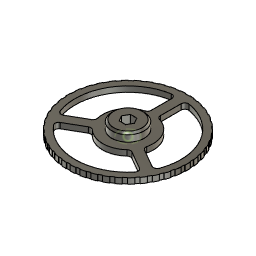
Flange gear v6 (Autodesk Fusion 360 design; units mm, degrees)
description: Spur Gear; Module: 2.0; Num Teeth: 10; Pressure Angle: 20.0; Backlash: 0.00 mm
Autodesk Fusion 360 part; units mm, degrees
(part 1 of 2)
sketch "Sketch1" plane through (0, 0, 0) normal (0, 0, 1) x (1, 0, 0) in component "Spur Gear (10 teeth)"
  circle A0 centre (0, 0) radius 7.5492
extrude "Extrude1" add sketch "Sketch1" along normal blind 7 makes body 1 in component "Spur Gear (10 teeth)"
sketch "Sketch2" plane through (0, 0, 0) normal (0, 0, 1) x (1, 0, 0) in component "Spur Gear (10 teeth)"
  spline S0 degree 5 poles (9.2583, -1.6082) (9.2659, -1.6095) (9.2813, -1.6119) (9.3043, -1.6147) (9.3352, -1.6169) (9.374, -1.6176) (9.4131, -1.6169) (9.4522, -1.6153) (9.4913, -1.6131) (9.5306, -1.6106) (9.5699, -1.6078) (9.6092, -1.6044) (9.6485, -1.6005) (9.688, -1.5957) (9.7275, -1.5903) (9.767, -1.5842) (9.8065, -1.5774) (9.8461, -1.5702) (9.8857, -1.5626) (9.9253, -1.5546) (9.9649, -1.5461) (10.0045, -1.5372) (10.0441, -1.5278) (10.0838, -1.5179) (10.1234, -1.5076) (10.163, -1.4969) (10.2027, -1.4857) (10.2423, -1.4741) (10.2819, -1.4621) (10.3215, -1.4497) (10.3611, -1.4369) (10.4006, -1.4237) (10.4402, -1.4102) (10.4797, -1.3962) (10.5192, -1.3819) (10.5587, -1.3672) (10.5982, -1.3521) (10.6376, -1.3367) (10.677, -1.3209) (10.7163, -1.3047) (10.7557, -1.2882) (10.795, -1.2713) (10.8342, -1.2541) (10.8734, -1.2366) (10.9126, -1.2187) (10.9517, -1.2004) (10.9908, -1.1818) (11.0298, -1.1629) (11.0688, -1.1437) (11.1078, -1.1241) (11.1466, -1.1042) (11.1855, -1.084) (11.2242, -1.0634) (11.2629, -1.0425) (11.3016, -1.0213) (11.3402, -0.9998) (11.3787, -0.978) (11.4172, -0.9559) (11.4556, -0.9334) (11.4939, -0.9107) (11.5322, -0.8876) (11.5704, -0.8642) (11.6085, -0.8406) (11.6466, -0.8166) (11.6846, -0.7923) (11.7225, -0.7677) (11.7603, -0.7429) (11.7981, -0.7177) (11.8358, -0.6923) (11.8733, -0.6665) (11.9109, -0.6405) (11.9408, -0.6194) (11.9632, -0.6035) (11.9781, -0.5928) (11.9856, -0.5875) knots 0 0 0 0 0 0 0.01428571 0.02857143 0.04285714 0.05714286 0.07142857 0.08571429 0.1 0.11428571 0.12857143 0.14285714 0.15714286 0.17142857 0.18571429 0.2 0.21428571 0.22857143 0.24285714 0.25714286 0.27142857 0.28571429 0.3 0.31428571 0.32857143 0.34285714 0.35714286 0.37142857 0.38571429 0.4 0.41428571 0.42857143 0.44285714 0.45714286 0.47142857 0.48571429 0.5 0.51428571 0.52857143 0.54285714 0.55714286 0.57142857 0.58571429 0.6 0.61428571 0.62857143 0.64285714 0.65714286 0.67142857 0.68571429 0.7 0.71428571 0.72857143 0.74285714 0.75714286 0.77142857 0.78571429 0.8 0.81428571 0.82857143 0.84285714 0.85714286 0.87142857 0.88571429 0.9 0.91428571 0.92857143 0.94285714 0.95714286 0.97142857 0.98571429 1 1 1 1 1 1
  spline S1 degree 5 poles (9.2583, 1.6082) (9.2659, 1.6095) (9.2813, 1.6119) (9.3043, 1.6147) (9.3352, 1.6169) (9.374, 1.6176) (9.4131, 1.6169) (9.4522, 1.6153) (9.4913, 1.6131) (9.5306, 1.6106) (9.5699, 1.6078) (9.6092, 1.6044) (9.6485, 1.6005) (9.688, 1.5957) (9.7275, 1.5903) (9.767, 1.5842) (9.8065, 1.5774) (9.8461, 1.5702) (9.8857, 1.5626) (9.9253, 1.5546) (9.9649, 1.5461) (10.0045, 1.5372) (10.0441, 1.5278) (10.0838, 1.5179) (10.1234, 1.5076) (10.163, 1.4969) (10.2027, 1.4857) (10.2423, 1.4741) (10.2819, 1.4621) (10.3215, 1.4497) (10.3611, 1.4369) (10.4006, 1.4237) (10.4402, 1.4102) (10.4797, 1.3962) (10.5192, 1.3819) (10.5587, 1.3672) (10.5982, 1.3521) (10.6376, 1.3367) (10.677, 1.3209) (10.7163, 1.3047) (10.7557, 1.2882) (10.795, 1.2713) (10.8342, 1.2541) (10.8734, 1.2366) (10.9126, 1.2187) (10.9517, 1.2004) (10.9908, 1.1818) (11.0298, 1.1629) (11.0688, 1.1437) (11.1078, 1.1241) (11.1466, 1.1042) (11.1855, 1.084) (11.2242, 1.0634) (11.2629, 1.0425) (11.3016, 1.0213) (11.3402, 0.9998) (11.3787, 0.978) (11.4172, 0.9559) (11.4556, 0.9334) (11.4939, 0.9107) (11.5322, 0.8876) (11.5704, 0.8642) (11.6085, 0.8406) (11.6466, 0.8166) (11.6846, 0.7923) (11.7225, 0.7677) (11.7603, 0.7429) (11.7981, 0.7177) (11.8358, 0.6923) (11.8733, 0.6665) (11.9109, 0.6405) (11.9408, 0.6194) (11.9632, 0.6035) (11.9781, 0.5928) (11.9856, 0.5875) knots 0 0 0 0 0 0 0.01428571 0.02857143 0.04285714 0.05714286 0.07142857 0.08571429 0.1 0.11428571 0.12857143 0.14285714 0.15714286 0.17142857 0.18571429 0.2 0.21428571 0.22857143 0.24285714 0.25714286 0.27142857 0.28571429 0.3 0.31428571 0.32857143 0.34285714 0.35714286 0.37142857 0.38571429 0.4 0.41428571 0.42857143 0.44285714 0.45714286 0.47142857 0.48571429 0.5 0.51428571 0.52857143 0.54285714 0.55714286 0.57142857 0.58571429 0.6 0.61428571 0.62857143 0.64285714 0.65714286 0.67142857 0.68571429 0.7 0.71428571 0.72857143 0.74285714 0.75714286 0.77142857 0.78571429 0.8 0.81428571 0.82857143 0.84285714 0.85714286 0.87142857 0.88571429 0.9 0.91428571 0.92857143 0.94285714 0.95714286 0.97142857 0.98571429 1 1 1 1 1 1
  arc A0 (11.9856, -0.5875) -> (11.9856, 0.5875) centre (0, 0) ccw
  line L0 (7.428, -1.292) -> (9.2583, -1.6082)
  line L1 (7.428, 1.292) -> (9.2583, 1.6082)
  line L2 (7.428, -1.292) -> (7.428, 1.292)
  point P0 (9.4457, -1.6154)
  point P1 (9.6366, -1.6016)
  point P2 (9.8296, -1.5732)
  point P3 (10.0242, -1.5325)
  point P4 (10.2199, -1.4806)
  point P5 (10.4164, -1.4183)
  point P6 (10.6134, -1.3461)
  point P7 (10.8107, -1.2644)
  point P8 (11.008, -1.1735)
  point P9 (11.205, -1.0736)
  point P10 (11.4014, -0.9649)
  point P11 (11.5972, -0.8476)
  point P12 (11.792, -0.7217)
  point P13 (9.4457, 1.6154)
  point P14 (9.6366, 1.6016)
  point P15 (9.8296, 1.5732)
  point P16 (10.0242, 1.5325)
  point P17 (10.2199, 1.4806)
  point P18 (10.4164, 1.4183)
  point P19 (10.6134, 1.3461)
  point P20 (10.8107, 1.2644)
  point P21 (11.008, 1.1735)
  point P22 (11.205, 1.0736)
  point P23 (11.4014, 0.9649)
  point P24 (11.5972, 0.8476)
  point P25 (11.792, 0.7217)
extrude "Extrude2" add sketch "Sketch2" along normal blind 7 bodies 1 in component "Spur Gear (10 teeth)"
fillet "Fillet1" radius 1 2 edges at (7.4375, -1.2936, 3.5) (7.4375, 1.2936, 3.5) on bodies 1 in component "Spur Gear (10 teeth)"
pattern_circular "C-Pattern1" count 10 over 360 about axis through (0, 0, 0) along (0, 0, 1) of "Extrude2", "Fillet1" in component "Spur Gear (10 teeth)"
sketch "Sketch3" plane through (0, 0, 0) normal (0, 0, 1) x (1, 0, 0) in component "Spur Gear (10 teeth)"
  circle A0 centre (0, 0) radius 10 construction
sketch "Sketch1 (2)" plane through (0, 0, 7) normal (0, 0, 1) x (-1, 0, 0)
  arc A0 (-7.1196, 2.5104) -> (-7.2354, 2.1538) centre (0, 0) ccw
  arc A1 (-8.3641, 1.4537) -> (-7.2354, 2.1538) centre (-8.1939, 2.4391) ccw
  line L0 (-8.3641, 1.4537) -> (-9.2583, 1.6082)
  spline S0 degree 5 poles (-9.2583, 1.6082) (-9.2659, 1.6095) (-9.2813, 1.6119) (-9.3043, 1.6147) (-9.3352, 1.6169) (-9.374, 1.6176) (-9.4131, 1.6169) (-9.4522, 1.6153) (-9.4913, 1.6131) (-9.5306, 1.6106) (-9.5699, 1.6078) (-9.6092, 1.6044) (-9.6485, 1.6005) (-9.688, 1.5957) (-9.7275, 1.5903) (-9.767, 1.5842) (-9.8065, 1.5774) (-9.8461, 1.5702) (-9.8857, 1.5626) (-9.9253, 1.5546) (-9.9649, 1.5461) (-10.0045, 1.5372) (-10.0441, 1.5278) (-10.0838, 1.5179) (-10.1234, 1.5076) (-10.163, 1.4969) (-10.2027, 1.4857) (-10.2423, 1.4741) (-10.2819, 1.4621) (-10.3215, 1.4497) (-10.3611, 1.4369) (-10.4006, 1.4237) (-10.4402, 1.4102) (-10.4797, 1.3962) (-10.5192, 1.3819) (-10.5587, 1.3672) (-10.5982, 1.3521) (-10.6376, 1.3367) (-10.677, 1.3209) (-10.7163, 1.3047) (-10.7557, 1.2882) (-10.795, 1.2713) (-10.8342, 1.2541) (-10.8734, 1.2366) (-10.9126, 1.2187) (-10.9517, 1.2004) (-10.9908, 1.1818) (-11.0298, 1.1629) (-11.0688, 1.1437) (-11.1078, 1.1241) (-11.1466, 1.1042) (-11.1855, 1.084) (-11.2242, 1.0634) (-11.2629, 1.0425) (-11.3016, 1.0213) (-11.3402, 0.9998) (-11.3787, 0.978) (-11.4172, 0.9559) (-11.4556, 0.9334) (-11.4939, 0.9107) (-11.5322, 0.8876) (-11.5704, 0.8642) (-11.6085, 0.8406) (-11.6466, 0.8166) (-11.6846, 0.7923) (-11.7225, 0.7677) (-11.7603, 0.7429) (-11.7981, 0.7177) (-11.8358, 0.6923) (-11.8733, 0.6665) (-11.9109, 0.6405) (-11.9408, 0.6194) (-11.9632, 0.6035) (-11.9781, 0.5928) (-11.9856, 0.5875) knots 0 0 0 0 0 0 0.01428571 0.02857143 0.04285714 0.05714286 0.07142857 0.08571429 0.1 0.11428571 0.12857143 0.14285714 0.15714286 0.17142857 0.18571429 0.2 0.21428571 0.22857143 0.24285714 0.25714286 0.27142857 0.28571429 0.3 0.31428571 0.32857143 0.34285714 0.35714286 0.37142857 0.38571429 0.4 0.41428571 0.42857143 0.44285714 0.45714286 0.47142857 0.48571429 0.5 0.51428571 0.52857143 0.54285714 0.55714286 0.57142857 0.58571429 0.6 0.61428571 0.62857143 0.64285714 0.65714286 0.67142857 0.68571429 0.7 0.71428571 0.72857143 0.74285714 0.75714286 0.77142857 0.78571429 0.8 0.81428571 0.82857143 0.84285714 0.85714286 0.87142857 0.88571429 0.9 0.91428571 0.92857143 0.94285714 0.95714286 0.97142857 0.98571429 1 1 1 1 1 1
  arc A2 (-11.9856, 0.5875) -> (-11.9856, -0.5875) centre (0, 0) ccw
  spline S1 degree 5 poles (-11.9856, -0.5875) (-11.9781, -0.5928) (-11.9632, -0.6035) (-11.9408, -0.6194) (-11.9109, -0.6405) (-11.8733, -0.6665) (-11.8358, -0.6923) (-11.7981, -0.7177) (-11.7603, -0.7429) (-11.7225, -0.7677) (-11.6846, -0.7923) (-11.6466, -0.8166) (-11.6085, -0.8406) (-11.5704, -0.8642) (-11.5322, -0.8876) (-11.4939, -0.9107) (-11.4556, -0.9334) (-11.4172, -0.9559) (-11.3787, -0.978) (-11.3402, -0.9998) (-11.3016, -1.0213) (-11.2629, -1.0425) (-11.2242, -1.0634) (-11.1855, -1.084) (-11.1466, -1.1042) (-11.1078, -1.1241) (-11.0688, -1.1437) (-11.0298, -1.1629) (-10.9908, -1.1818) (-10.9517, -1.2004) (-10.9126, -1.2187) (-10.8734, -1.2366) (-10.8342, -1.2541) (-10.795, -1.2713) (-10.7557, -1.2882) (-10.7163, -1.3047) (-10.677, -1.3209) (-10.6376, -1.3367) (-10.5982, -1.3521) (-10.5587, -1.3672) (-10.5192, -1.3819) (-10.4797, -1.3962) (-10.4402, -1.4102) (-10.4006, -1.4237) (-10.3611, -1.4369) (-10.3215, -1.4497) (-10.2819, -1.4621) (-10.2423, -1.4741) (-10.2027, -1.4857) (-10.163, -1.4969) (-10.1234, -1.5076) (-10.0838, -1.5179) (-10.0441, -1.5278) (-10.0045, -1.5372) (-9.9649, -1.5461) (-9.9253, -1.5546) (-9.8857, -1.5626) (-9.8461, -1.5702) (-9.8065, -1.5774) (-9.767, -1.5842) (-9.7275, -1.5903) (-9.688, -1.5957) (-9.6485, -1.6005) (-9.6092, -1.6044) (-9.5699, -1.6078) (-9.5306, -1.6106) (-9.4913, -1.6131) (-9.4522, -1.6153) (-9.4131, -1.6169) (-9.374, -1.6176) (-9.3352, -1.6169) (-9.3043, -1.6147) (-9.2813, -1.6119) (-9.2659, -1.6095) (-9.2583, -1.6082) knots -1 -1 -1 -1 -1 -1 -0.98571429 -0.97142857 -0.95714286 -0.94285714 -0.92857143 -0.91428571 -0.9 -0.88571429 -0.87142857 -0.85714286 -0.84285714 -0.82857143 -0.81428571 -0.8 -0.78571429 -0.77142857 -0.75714286 -0.74285714 -0.72857143 -0.71428571 -0.7 -0.68571429 -0.67142857 -0.65714286 -0.64285714 -0.62857143 -0.61428571 -0.6 -0.58571429 -0.57142857 -0.55714286 -0.54285714 -0.52857143 -0.51428571 -0.5 -0.48571429 -0.47142857 -0.45714286 -0.44285714 -0.42857143 -0.41428571 -0.4 -0.38571429 -0.37142857 -0.35714286 -0.34285714 -0.32857143 -0.31428571 -0.3 -0.28571429 -0.27142857 -0.25714286 -0.24285714 -0.22857143 -0.21428571 -0.2 -0.18571429 -0.17142857 -0.15714286 -0.14285714 -0.12857143 -0.11428571 -0.1 -0.08571429 -0.07142857 -0.05714286 -0.04285714 -0.02857143 -0.01428571 0 0 0 0 0 0
  line L1 (-9.2583, -1.6082) -> (-8.3641, -1.4537)
  arc A3 (-7.2354, -2.1538) -> (-8.3641, -1.4537) centre (-8.1939, -2.4391) ccw
  arc A4 (-7.2354, -2.1538) -> (-7.1196, -2.5104) centre (0, 0) ccw
  arc A5 (-7.6212, -3.7403) -> (-7.1196, -2.5104) centre (-8.0626, -2.843) ccw
  line L2 (-7.6212, -3.7403) -> (-8.4354, -4.1409)
  spline S2 degree 5 poles (-8.4354, -4.1409) (-8.4423, -4.1443) (-8.4561, -4.1514) (-8.4764, -4.1627) (-8.5027, -4.179) (-8.5346, -4.2013) (-8.5657, -4.2248) (-8.5964, -4.2491) (-8.6268, -4.2738) (-8.6571, -4.2989) (-8.6872, -4.3243) (-8.7171, -4.3501) (-8.7466, -4.3765) (-8.7757, -4.4035) (-8.8044, -4.4311) (-8.8328, -4.4593) (-8.8608, -4.4879) (-8.8886, -4.517) (-8.9162, -4.5465) (-8.9435, -4.5763) (-8.9705, -4.6064) (-8.9973, -4.6369) (-9.0239, -4.6678) (-9.0502, -4.699) (-9.0762, -4.7307) (-9.1019, -4.7627) (-9.1274, -4.795) (-9.1526, -4.8277) (-9.1776, -4.8607) (-9.2024, -4.894) (-9.2269, -4.9276) (-9.2511, -4.9615) (-9.2752, -4.9957) (-9.299, -5.0303) (-9.3225, -5.0651) (-9.3458, -5.1002) (-9.3688, -5.1356) (-9.3917, -5.1712) (-9.4142, -5.2072) (-9.4366, -5.2434) (-9.4587, -5.2799) (-9.4806, -5.3166) (-9.5022, -5.3536) (-9.5236, -5.3908) (-9.5448, -5.4283) (-9.5657, -5.4661) (-9.5864, -5.5041) (-9.6069, -5.5424) (-9.6271, -5.5808) (-9.6471, -5.6196) (-9.6668, -5.6585) (-9.6864, -5.6977) (-9.7056, -5.7371) (-9.7247, -5.7768) (-9.7435, -5.8166) (-9.7621, -5.8567) (-9.7804, -5.897) (-9.7986, -5.9376) (-9.8164, -5.9783) (-9.8341, -6.0192) (-9.8515, -6.0604) (-9.8686, -6.1017) (-9.8856, -6.1433) (-9.9023, -6.1851) (-9.9187, -6.227) (-9.935, -6.2692) (-9.951, -6.3115) (-9.9667, -6.3541) (-9.9822, -6.3968) (-9.9975, -6.4398) (-10.0126, -6.4829) (-10.0244, -6.5175) (-10.0332, -6.5436) (-10.039, -6.561) (-10.0419, -6.5697) knots 0 0 0 0 0 0 0.01428571 0.02857143 0.04285714 0.05714286 0.07142857 0.08571429 0.1 0.11428571 0.12857143 0.14285714 0.15714286 0.17142857 0.18571429 0.2 0.21428571 0.22857143 0.24285714 0.25714286 0.27142857 0.28571429 0.3 0.31428571 0.32857143 0.34285714 0.35714286 0.37142857 0.38571429 0.4 0.41428571 0.42857143 0.44285714 0.45714286 0.47142857 0.48571429 0.5 0.51428571 0.52857143 0.54285714 0.55714286 0.57142857 0.58571429 0.6 0.61428571 0.62857143 0.64285714 0.65714286 0.67142857 0.68571429 0.7 0.71428571 0.72857143 0.74285714 0.75714286 0.77142857 0.78571429 0.8 0.81428571 0.82857143 0.84285714 0.85714286 0.87142857 0.88571429 0.9 0.91428571 0.92857143 0.94285714 0.95714286 0.97142857 0.98571429 1 1 1 1 1 1
  arc A6 (-10.0419, -6.5697) -> (-9.3513, -7.5202) centre (0, 0) ccw
  spline S3 degree 5 poles (-9.3513, -7.5202) (-9.3421, -7.5202) (-9.3237, -7.52) (-9.2962, -7.5198) (-9.2596, -7.5192) (-9.214, -7.5182) (-9.1684, -7.5169) (-9.123, -7.5154) (-9.0777, -7.5136) (-9.0324, -7.5114) (-8.9873, -7.509) (-8.9423, -7.5063) (-8.8974, -7.5034) (-8.8527, -7.5001) (-8.808, -7.4965) (-8.7635, -7.4927) (-8.7191, -7.4886) (-8.6749, -7.4842) (-8.6307, -7.4795) (-8.5867, -7.4745) (-8.5429, -7.4692) (-8.4991, -7.4636) (-8.4555, -7.4577) (-8.4121, -7.4516) (-8.3688, -7.4451) (-8.3256, -7.4384) (-8.2826, -7.4313) (-8.2398, -7.424) (-8.1971, -7.4164) (-8.1545, -7.4084) (-8.1122, -7.4002) (-8.07, -7.3916) (-8.0279, -7.3828) (-7.986, -7.3737) (-7.9443, -7.3642) (-7.9028, -7.3544) (-7.8615, -7.3444) (-7.8203, -7.334) (-7.7793, -7.3233) (-7.7386, -7.3123) (-7.698, -7.301) (-7.6576, -7.2894) (-7.6174, -7.2774) (-7.5775, -7.2652) (-7.5377, -7.2526) (-7.4982, -7.2396) (-7.4588, -7.2264) (-7.4197, -7.2128) (-7.3809, -7.1989) (-7.3422, -7.1847) (-7.3038, -7.1701) (-7.2657, -7.1551) (-7.2279, -7.1398) (-7.1903, -7.1241) (-7.153, -7.108) (-7.116, -7.0916) (-7.0792, -7.0748) (-7.0427, -7.0577) (-7.0064, -7.0403) (-6.9705, -7.0225) (-6.9349, -7.0042) (-6.8998, -6.9854) (-6.8651, -6.9661) (-6.8309, -6.9462) (-6.7971, -6.9257) (-6.7637, -6.905) (-6.7305, -6.8839) (-6.6975, -6.8626) (-6.6649, -6.8409) (-6.633, -6.8186) (-6.602, -6.7952) (-6.5783, -6.7752) (-6.5613, -6.7594) (-6.5503, -6.7485) (-6.5449, -6.7429) knots -1 -1 -1 -1 -1 -1 -0.98571429 -0.97142857 -0.95714286 -0.94285714 -0.92857143 -0.91428571 -0.9 -0.88571429 -0.87142857 -0.85714286 -0.84285714 -0.82857143 -0.81428571 -0.8 -0.78571429 -0.77142857 -0.75714286 -0.74285714 -0.72857143 -0.71428571 -0.7 -0.68571429 -0.67142857 -0.65714286 -0.64285714 -0.62857143 -0.61428571 -0.6 -0.58571429 -0.57142857 -0.55714286 -0.54285714 -0.52857143 -0.51428571 -0.5 -0.48571429 -0.47142857 -0.45714286 -0.44285714 -0.42857143 -0.41428571 -0.4 -0.38571429 -0.37142857 -0.35714286 -0.34285714 -0.32857143 -0.31428571 -0.3 -0.28571429 -0.27142857 -0.25714286 -0.24285714 -0.22857143 -0.21428571 -0.2 -0.18571429 -0.17142857 -0.15714286 -0.14285714 -0.12857143 -0.11428571 -0.1 -0.08571429 -0.07142857 -0.05714286 -0.04285714 -0.02857143 -0.01428571 0 0 0 0 0 0
  line L3 (-6.5449, -6.7429) -> (-5.9123, -6.0924)
  arc A7 (-4.5876, -5.9953) -> (-5.9123, -6.0924) centre (-5.1953, -6.7895) ccw
  arc A8 (-4.5876, -5.9953) -> (-4.2842, -6.2158) centre (0, 0) ccw
  arc A9 (-3.9672, -7.5055) -> (-4.2842, -6.2158) centre (-4.8518, -7.0391) ccw
  line L4 (-3.9672, -7.5055) -> (-4.3904, -8.3082)
  spline S4 degree 5 poles (-4.3904, -8.3082) (-4.394, -8.3151) (-4.401, -8.3289) (-4.4108, -8.35) (-4.4225, -8.3787) (-4.4352, -8.4154) (-4.4465, -8.4527) (-4.4571, -8.4904) (-4.4672, -8.5283) (-4.4769, -8.5664) (-4.4863, -8.6046) (-4.4953, -8.6431) (-4.5037, -8.6817) (-4.5114, -8.7207) (-4.5184, -8.7599) (-4.5248, -8.7994) (-4.5306, -8.8391) (-4.536, -8.879) (-4.541, -8.919) (-4.5455, -8.9591) (-4.5497, -8.9994) (-4.5535, -9.0398) (-4.5568, -9.0804) (-4.5597, -9.1212) (-4.5621, -9.162) (-4.5641, -9.2031) (-4.5657, -9.2442) (-4.567, -9.2855) (-4.5678, -9.3269) (-4.5682, -9.3683) (-4.5683, -9.4099) (-4.568, -9.4516) (-4.5673, -9.4934) (-4.5663, -9.5353) (-4.5649, -9.5773) (-4.5631, -9.6194) (-4.5609, -9.6616) (-4.5584, -9.7039) (-4.5556, -9.7462) (-4.5524, -9.7887) (-4.5488, -9.8312) (-4.5449, -9.8738) (-4.5407, -9.9164) (-4.5361, -9.9591) (-4.5312, -10.0019) (-4.5259, -10.0448) (-4.5203, -10.0877) (-4.5144, -10.1306) (-4.5081, -10.1737) (-4.5016, -10.2167) (-4.4946, -10.2599) (-4.4874, -10.303) (-4.4798, -10.3463) (-4.4719, -10.3895) (-4.4637, -10.4329) (-4.4552, -10.4762) (-4.4464, -10.5196) (-4.4372, -10.563) (-4.4277, -10.6065) (-4.4179, -10.65) (-4.4078, -10.6935) (-4.3974, -10.7371) (-4.3867, -10.7806) (-4.3756, -10.8242) (-4.3643, -10.8679) (-4.3526, -10.9115) (-4.3407, -10.9552) (-4.3284, -10.9989) (-4.3158, -11.0426) (-4.303, -11.0863) (-4.2898, -11.13) (-4.279, -11.165) (-4.2708, -11.1912) (-4.2653, -11.2087) (-4.2625, -11.2175) knots 0 0 0 0 0 0 0.01428571 0.02857143 0.04285714 0.05714286 0.07142857 0.08571429 0.1 0.11428571 0.12857143 0.14285714 0.15714286 0.17142857 0.18571429 0.2 0.21428571 0.22857143 0.24285714 0.25714286 0.27142857 0.28571429 0.3 0.31428571 0.32857143 0.34285714 0.35714286 0.37142857 0.38571429 0.4 0.41428571 0.42857143 0.44285714 0.45714286 0.47142857 0.48571429 0.5 0.51428571 0.52857143 0.54285714 0.55714286 0.57142857 0.58571429 0.6 0.61428571 0.62857143 0.64285714 0.65714286 0.67142857 0.68571429 0.7 0.71428571 0.72857143 0.74285714 0.75714286 0.77142857 0.78571429 0.8 0.81428571 0.82857143 0.84285714 0.85714286 0.87142857 0.88571429 0.9 0.91428571 0.92857143 0.94285714 0.95714286 0.97142857 0.98571429 1 1 1 1 1 1
  arc A10 (-4.2625, -11.2175) -> (-3.145, -11.5805) centre (0, 0) ccw
  spline S5 degree 5 poles (-3.145, -11.5805) (-3.1376, -11.5751) (-3.1229, -11.5642) (-3.1008, -11.5478) (-3.0715, -11.5258) (-3.0352, -11.4982) (-2.9991, -11.4704) (-2.9632, -11.4424) (-2.9276, -11.4143) (-2.8923, -11.386) (-2.8572, -11.3575) (-2.8224, -11.3289) (-2.7878, -11.3001) (-2.7535, -11.2712) (-2.7195, -11.2421) (-2.6857, -11.2128) (-2.6522, -11.1834) (-2.619, -11.1538) (-2.5861, -11.124) (-2.5534, -11.0941) (-2.521, -11.0641) (-2.4889, -11.0339) (-2.4571, -11.0035) (-2.4256, -10.973) (-2.3944, -10.9423) (-2.3634, -10.9115) (-2.3328, -10.8805) (-2.3024, -10.8494) (-2.2724, -10.8181) (-2.2426, -10.7867) (-2.2132, -10.7551) (-2.184, -10.7234) (-2.1552, -10.6915) (-2.1267, -10.6595) (-2.0985, -10.6273) (-2.0707, -10.595) (-2.0431, -10.5626) (-2.0159, -10.53) (-1.9891, -10.4973) (-1.9625, -10.4644) (-1.9364, -10.4314) (-1.9105, -10.3983) (-1.885, -10.365) (-1.8599, -10.3316) (-1.8352, -10.298) (-1.8108, -10.2643) (-1.7868, -10.2305) (-1.7631, -10.1965) (-1.7398, -10.1624) (-1.7169, -10.1282) (-1.6945, -10.0938) (-1.6724, -10.0593) (-1.6508, -10.0246) (-1.6296, -9.9899) (-1.6089, -9.9549) (-1.5886, -9.9199) (-1.5687, -9.8847) (-1.5492, -9.8494) (-1.5301, -9.814) (-1.5115, -9.7785) (-1.4935, -9.7428) (-1.4761, -9.7069) (-1.4594, -9.6709) (-1.4435, -9.6347) (-1.4282, -9.5983) (-1.4133, -9.5618) (-1.3988, -9.5253) (-1.3847, -9.4887) (-1.371, -9.452) (-1.3583, -9.4151) (-1.347, -9.378) (-1.3396, -9.3479) (-1.3351, -9.3251) (-1.3326, -9.3098) (-1.3315, -9.3021) knots -1 -1 -1 -1 -1 -1 -0.98571429 -0.97142857 -0.95714286 -0.94285714 -0.92857143 -0.91428571 -0.9 -0.88571429 -0.87142857 -0.85714286 -0.84285714 -0.82857143 -0.81428571 -0.8 -0.78571429 -0.77142857 -0.75714286 -0.74285714 -0.72857143 -0.71428571 -0.7 -0.68571429 -0.67142857 -0.65714286 -0.64285714 -0.62857143 -0.61428571 -0.6 -0.58571429 -0.57142857 -0.55714286 -0.54285714 -0.52857143 -0.51428571 -0.5 -0.48571429 -0.47142857 -0.45714286 -0.44285714 -0.42857143 -0.41428571 -0.4 -0.38571429 -0.37142857 -0.35714286 -0.34285714 -0.32857143 -0.31428571 -0.3 -0.28571429 -0.27142857 -0.25714286 -0.24285714 -0.22857143 -0.21428571 -0.2 -0.18571429 -0.17142857 -0.15714286 -0.14285714 -0.12857143 -0.11428571 -0.1 -0.08571429 -0.07142857 -0.05714286 -0.04285714 -0.02857143 -0.01428571 0 0 0 0 0 0
  line L5 (-1.3315, -9.3021) -> (-1.2021, -8.404)
  arc A11 (-0.1875, -7.5469) -> (-1.2021, -8.404) centre (-0.2123, -8.5466) ccw
  arc A12 (-0.1875, -7.5469) -> (0.1875, -7.5469) centre (0, 0) ccw
  arc A13 (1.2021, -8.404) -> (0.1875, -7.5469) centre (0.2123, -8.5466) ccw
  line L6 (1.2021, -8.404) -> (1.3315, -9.3021)
  spline S6 degree 5 poles (1.3315, -9.3021) (1.3326, -9.3098) (1.3351, -9.3251) (1.3396, -9.3479) (1.347, -9.378) (1.3583, -9.4151) (1.371, -9.452) (1.3847, -9.4887) (1.3988, -9.5253) (1.4133, -9.5618) (1.4282, -9.5983) (1.4435, -9.6347) (1.4594, -9.6709) (1.4761, -9.7069) (1.4935, -9.7428) (1.5115, -9.7785) (1.5301, -9.814) (1.5492, -9.8494) (1.5687, -9.8847) (1.5886, -9.9199) (1.6089, -9.9549) (1.6296, -9.9899) (1.6508, -10.0246) (1.6724, -10.0593) (1.6945, -10.0938) (1.7169, -10.1282) (1.7398, -10.1624) (1.7631, -10.1965) (1.7868, -10.2305) (1.8108, -10.2643) (1.8352, -10.298) (1.8599, -10.3316) (1.885, -10.365) (1.9105, -10.3983) (1.9364, -10.4314) (1.9625, -10.4644) (1.9891, -10.4973) (2.0159, -10.53) (2.0431, -10.5626) (2.0707, -10.595) (2.0985, -10.6273) (2.1267, -10.6595) (2.1552, -10.6915) (2.184, -10.7234) (2.2132, -10.7551) (2.2426, -10.7867) (2.2724, -10.8181) (2.3024, -10.8494) (2.3328, -10.8805) (2.3634, -10.9115) (2.3944, -10.9423) (2.4256, -10.973) (2.4571, -11.0035) (2.4889, -11.0339) (2.521, -11.0641) (2.5534, -11.0941) (2.5861, -11.124) (2.619, -11.1538) (2.6522, -11.1834) (2.6857, -11.2128) (2.7195, -11.2421) (2.7535, -11.2712) (2.7878, -11.3001) (2.8224, -11.3289) (2.8572, -11.3575) (2.8923, -11.386) (2.9276, -11.4143) (2.9632, -11.4424) (2.9991, -11.4704) (3.0352, -11.4982) (3.0715, -11.5258) (3.1008, -11.5478) (3.1229, -11.5642) (3.1376, -11.5751) (3.145, -11.5805) knots 0 0 0 0 0 0 0.01428571 0.02857143 0.04285714 0.05714286 0.07142857 0.08571429 0.1 0.11428571 0.12857143 0.14285714 0.15714286 0.17142857 0.18571429 0.2 0.21428571 0.22857143 0.24285714 0.25714286 0.27142857 0.28571429 0.3 0.31428571 0.32857143 0.34285714 0.35714286 0.37142857 0.38571429 0.4 0.41428571 0.42857143 0.44285714 0.45714286 0.47142857 0.48571429 0.5 0.51428571 0.52857143 0.54285714 0.55714286 0.57142857 0.58571429 0.6 0.61428571 0.62857143 0.64285714 0.65714286 0.67142857 0.68571429 0.7 0.71428571 0.72857143 0.74285714 0.75714286 0.77142857 0.78571429 0.8 0.81428571 0.82857143 0.84285714 0.85714286 0.87142857 0.88571429 0.9 0.91428571 0.92857143 0.94285714 0.95714286 0.97142857 0.98571429 1 1 1 1 1 1
  arc A14 (3.145, -11.5805) -> (4.2625, -11.2175) centre (0, 0) ccw
  spline S7 degree 5 poles (4.2625, -11.2175) (4.2653, -11.2087) (4.2708, -11.1912) (4.279, -11.165) (4.2898, -11.13) (4.303, -11.0863) (4.3158, -11.0426) (4.3284, -10.9989) (4.3407, -10.9552) (4.3526, -10.9115) (4.3643, -10.8679) (4.3756, -10.8242) (4.3867, -10.7806) (4.3974, -10.7371) (4.4078, -10.6935) (4.4179, -10.65) (4.4277, -10.6065) (4.4372, -10.563) (4.4464, -10.5196) (4.4552, -10.4762) (4.4637, -10.4329) (4.4719, -10.3895) (4.4798, -10.3463) (4.4874, -10.303) (4.4946, -10.2599) (4.5016, -10.2167) (4.5081, -10.1737) (4.5144, -10.1306) (4.5203, -10.0877) (4.5259, -10.0448) (4.5312, -10.0019) (4.5361, -9.9591) (4.5407, -9.9164) (4.5449, -9.8738) (4.5488, -9.8312) (4.5524, -9.7887) (4.5556, -9.7462) (4.5584, -9.7039) (4.5609, -9.6616) (4.5631, -9.6194) (4.5649, -9.5773) (4.5663, -9.5353) (4.5673, -9.4934) (4.568, -9.4516) (4.5683, -9.4099) (4.5682, -9.3683) (4.5678, -9.3269) (4.567, -9.2855) (4.5657, -9.2442) (4.5641, -9.2031) (4.5621, -9.162) (4.5597, -9.1212) (4.5568, -9.0804) (4.5535, -9.0398) (4.5497, -8.9994) (4.5455, -8.9591) (4.541, -8.919) (4.536, -8.879) (4.5306, -8.8391) (4.5248, -8.7994) (4.5184, -8.7599) (4.5114, -8.7207) (4.5037, -8.6817) (4.4953, -8.6431) (4.4863, -8.6046) (4.4769, -8.5664) (4.4672, -8.5283) (4.4571, -8.4904) (4.4465, -8.4527) (4.4352, -8.4154) (4.4225, -8.3787) (4.4108, -8.35) (4.401, -8.3289) (4.394, -8.3151) (4.3904, -8.3082) knots -1 -1 -1 -1 -1 -1 -0.98571429 -0.97142857 -0.95714286 -0.94285714 -0.92857143 -0.91428571 -0.9 -0.88571429 -0.87142857 -0.85714286 -0.84285714 -0.82857143 -0.81428571 -0.8 -0.78571429 -0.77142857 -0.75714286 -0.74285714 -0.72857143 -0.71428571 -0.7 -0.68571429 -0.67142857 -0.65714286 -0.64285714 -0.62857143 -0.61428571 -0.6 -0.58571429 -0.57142857 -0.55714286 -0.54285714 -0.52857143 -0.51428571 -0.5 -0.48571429 -0.47142857 -0.45714286 -0.44285714 -0.42857143 -0.41428571 -0.4 -0.38571429 -0.37142857 -0.35714286 -0.34285714 -0.32857143 -0.31428571 -0.3 -0.28571429 -0.27142857 -0.25714286 -0.24285714 -0.22857143 -0.21428571 -0.2 -0.18571429 -0.17142857 -0.15714286 -0.14285714 -0.12857143 -0.11428571 -0.1 -0.08571429 -0.07142857 -0.05714286 -0.04285714 -0.02857143 -0.01428571 0 0 0 0 0 0
  line L7 (4.3904, -8.3082) -> (3.9672, -7.5055)
  arc A15 (4.2842, -6.2158) -> (3.9672, -7.5055) centre (4.8518, -7.0391) ccw
  arc A16 (4.2842, -6.2158) -> (4.5876, -5.9953) centre (0, 0) ccw
  arc A17 (5.9123, -6.0924) -> (4.5876, -5.9953) centre (5.1953, -6.7895) ccw
  line L8 (5.9123, -6.0924) -> (6.5449, -6.7429)
  spline S8 degree 5 poles (6.5449, -6.7429) (6.5503, -6.7485) (6.5613, -6.7594) (6.5783, -6.7752) (6.602, -6.7952) (6.633, -6.8186) (6.6649, -6.8409) (6.6975, -6.8626) (6.7305, -6.8839) (6.7637, -6.905) (6.7971, -6.9257) (6.8309, -6.9462) (6.8651, -6.9661) (6.8998, -6.9854) (6.9349, -7.0042) (6.9705, -7.0225) (7.0064, -7.0403) (7.0427, -7.0577) (7.0792, -7.0748) (7.116, -7.0916) (7.153, -7.108) (7.1903, -7.1241) (7.2279, -7.1398) (7.2657, -7.1551) (7.3038, -7.1701) (7.3422, -7.1847) (7.3809, -7.1989) (7.4197, -7.2128) (7.4588, -7.2264) (7.4982, -7.2396) (7.5377, -7.2526) (7.5775, -7.2652) (7.6174, -7.2774) (7.6576, -7.2894) (7.698, -7.301) (7.7386, -7.3123) (7.7793, -7.3233) (7.8203, -7.334) (7.8615, -7.3444) (7.9028, -7.3544) (7.9443, -7.3642) (7.986, -7.3737) (8.0279, -7.3828) (8.07, -7.3916) (8.1122, -7.4002) (8.1545, -7.4084) (8.1971, -7.4164) (8.2398, -7.424) (8.2826, -7.4313) (8.3256, -7.4384) (8.3688, -7.4451) (8.4121, -7.4516) (8.4555, -7.4577) (8.4991, -7.4636) (8.5429, -7.4692) (8.5867, -7.4745) (8.6307, -7.4795) (8.6749, -7.4842) (8.7191, -7.4886) (8.7635, -7.4927) (8.808, -7.4965) (8.8527, -7.5001) (8.8974, -7.5034) (8.9423, -7.5063) (8.9873, -7.509) (9.0324, -7.5114) (9.0777, -7.5136) (9.123, -7.5154) (9.1684, -7.5169) (9.214, -7.5182) (9.2596, -7.5192) (9.2962, -7.5198) (9.3237, -7.52) (9.3421, -7.5202) (9.3513, -7.5202) knots 0 0 0 0 0 0 0.01428571 0.02857143 0.04285714 0.05714286 0.07142857 0.08571429 0.1 0.11428571 0.12857143 0.14285714 0.15714286 0.17142857 0.18571429 0.2 0.21428571 0.22857143 0.24285714 0.25714286 0.27142857 0.28571429 0.3 0.31428571 0.32857143 0.34285714 0.35714286 0.37142857 0.38571429 0.4 0.41428571 0.42857143 0.44285714 0.45714286 0.47142857 0.48571429 0.5 0.51428571 0.52857143 0.54285714 0.55714286 0.57142857 0.58571429 0.6 0.61428571 0.62857143 0.64285714 0.65714286 0.67142857 0.68571429 0.7 0.71428571 0.72857143 0.74285714 0.75714286 0.77142857 0.78571429 0.8 0.81428571 0.82857143 0.84285714 0.85714286 0.87142857 0.88571429 0.9 0.91428571 0.92857143 0.94285714 0.95714286 0.97142857 0.98571429 1 1 1 1 1 1
  arc A18 (9.3513, -7.5202) -> (10.0419, -6.5697) centre (0, 0) ccw
  spline S9 degree 5 poles (10.0419, -6.5697) (10.039, -6.561) (10.0332, -6.5436) (10.0244, -6.5175) (10.0126, -6.4829) (9.9975, -6.4398) (9.9822, -6.3968) (9.9667, -6.3541) (9.951, -6.3115) (9.935, -6.2692) (9.9187, -6.227) (9.9023, -6.1851) (9.8856, -6.1433) (9.8686, -6.1017) (9.8515, -6.0604) (9.8341, -6.0192) (9.8164, -5.9783) (9.7986, -5.9376) (9.7804, -5.897) (9.7621, -5.8567) (9.7435, -5.8166) (9.7247, -5.7768) (9.7056, -5.7371) (9.6864, -5.6977) (9.6668, -5.6585) (9.6471, -5.6196) (9.6271, -5.5808) (9.6069, -5.5424) (9.5864, -5.5041) (9.5657, -5.4661) (9.5448, -5.4283) (9.5236, -5.3908) (9.5022, -5.3536) (9.4806, -5.3166) (9.4587, -5.2799) (9.4366, -5.2434) (9.4142, -5.2072) (9.3917, -5.1712) (9.3688, -5.1356) (9.3458, -5.1002) (9.3225, -5.0651) (9.299, -5.0303) (9.2752, -4.9957) (9.2511, -4.9615) (9.2269, -4.9276) (9.2024, -4.894) (9.1776, -4.8607) (9.1526, -4.8277) (9.1274, -4.795) (9.1019, -4.7627) (9.0762, -4.7307) (9.0502, -4.699) (9.0239, -4.6678) (8.9973, -4.6369) (8.9705, -4.6064) (8.9435, -4.5763) (8.9162, -4.5465) (8.8886, -4.517) (8.8608, -4.4879) (8.8328, -4.4593) (8.8044, -4.4311) (8.7757, -4.4035) (8.7466, -4.3765) (8.7171, -4.3501) (8.6872, -4.3243) (8.6571, -4.2989) (8.6268, -4.2738) (8.5964, -4.2491) (8.5657, -4.2248) (8.5346, -4.2013) (8.5027, -4.179) (8.4764, -4.1627) (8.4561, -4.1514) (8.4423, -4.1443) (8.4354, -4.1409) knots -1 -1 -1 -1 -1 -1 -0.98571429 -0.97142857 -0.95714286 -0.94285714 -0.92857143 -0.91428571 -0.9 -0.88571429 -0.87142857 -0.85714286 -0.84285714 -0.82857143 -0.81428571 -0.8 -0.78571429 -0.77142857 -0.75714286 -0.74285714 -0.72857143 -0.71428571 -0.7 -0.68571429 -0.67142857 -0.65714286 -0.64285714 -0.62857143 -0.61428571 -0.6 -0.58571429 -0.57142857 -0.55714286 -0.54285714 -0.52857143 -0.51428571 -0.5 -0.48571429 -0.47142857 -0.45714286 -0.44285714 -0.42857143 -0.41428571 -0.4 -0.38571429 -0.37142857 -0.35714286 -0.34285714 -0.32857143 -0.31428571 -0.3 -0.28571429 -0.27142857 -0.25714286 -0.24285714 -0.22857143 -0.21428571 -0.2 -0.18571429 -0.17142857 -0.15714286 -0.14285714 -0.12857143 -0.11428571 -0.1 -0.08571429 -0.07142857 -0.05714286 -0.04285714 -0.02857143 -0.01428571 0 0 0 0 0 0
  line L9 (8.4354, -4.1409) -> (7.6212, -3.7403)
  arc A19 (7.1196, -2.5104) -> (7.6212, -3.7403) centre (8.0626, -2.843) ccw
  arc A20 (7.1196, -2.5104) -> (7.2354, -2.1538) centre (0, 0) ccw
  arc A21 (8.3641, -1.4537) -> (7.2354, -2.1538) centre (8.1939, -2.4391) ccw
  line L10 (8.3641, -1.4537) -> (9.2583, -1.6082)
  spline S10 degree 5 poles (9.2583, -1.6082) (9.2659, -1.6095) (9.2813, -1.6119) (9.3043, -1.6147) (9.3352, -1.6169) (9.374, -1.6176) (9.4131, -1.6169) (9.4522, -1.6153) (9.4913, -1.6131) (9.5306, -1.6106) (9.5699, -1.6078) (9.6092, -1.6044) (9.6485, -1.6005) (9.688, -1.5957) (9.7275, -1.5903) (9.767, -1.5842) (9.8065, -1.5774) (9.8461, -1.5702) (9.8857, -1.5626) (9.9253, -1.5546) (9.9649, -1.5461) (10.0045, -1.5372) (10.0441, -1.5278) (10.0838, -1.5179) (10.1234, -1.5076) (10.163, -1.4969) (10.2027, -1.4857) (10.2423, -1.4741) (10.2819, -1.4621) (10.3215, -1.4497) (10.3611, -1.4369) (10.4006, -1.4237) (10.4402, -1.4102) (10.4797, -1.3962) (10.5192, -1.3819) (10.5587, -1.3672) (10.5982, -1.3521) (10.6376, -1.3367) (10.677, -1.3209) (10.7163, -1.3047) (10.7557, -1.2882) (10.795, -1.2713) (10.8342, -1.2541) (10.8734, -1.2366) (10.9126, -1.2187) (10.9517, -1.2004) (10.9908, -1.1818) (11.0298, -1.1629) (11.0688, -1.1437) (11.1078, -1.1241) (11.1466, -1.1042) (11.1855, -1.084) (11.2242, -1.0634) (11.2629, -1.0425) (11.3016, -1.0213) (11.3402, -0.9998) (11.3787, -0.978) (11.4172, -0.9559) (11.4556, -0.9334) (11.4939, -0.9107) (11.5322, -0.8876) (11.5704, -0.8642) (11.6085, -0.8406) (11.6466, -0.8166) (11.6846, -0.7923) (11.7225, -0.7677) (11.7603, -0.7429) (11.7981, -0.7177) (11.8358, -0.6923) (11.8733, -0.6665) (11.9109, -0.6405) (11.9408, -0.6194) (11.9632, -0.6035) (11.9781, -0.5928) (11.9856, -0.5875) knots 0 0 0 0 0 0 0.01428571 0.02857143 0.04285714 0.05714286 0.07142857 0.08571429 0.1 0.11428571 0.12857143 0.14285714 0.15714286 0.17142857 0.18571429 0.2 0.21428571 0.22857143 0.24285714 0.25714286 0.27142857 0.28571429 0.3 0.31428571 0.32857143 0.34285714 0.35714286 0.37142857 0.38571429 0.4 0.41428571 0.42857143 0.44285714 0.45714286 0.47142857 0.48571429 0.5 0.51428571 0.52857143 0.54285714 0.55714286 0.57142857 0.58571429 0.6 0.61428571 0.62857143 0.64285714 0.65714286 0.67142857 0.68571429 0.7 0.71428571 0.72857143 0.74285714 0.75714286 0.77142857 0.78571429 0.8 0.81428571 0.82857143 0.84285714 0.85714286 0.87142857 0.88571429 0.9 0.91428571 0.92857143 0.94285714 0.95714286 0.97142857 0.98571429 1 1 1 1 1 1
  arc A22 (11.9856, -0.5875) -> (11.9856, 0.5875) centre (0, 0) ccw
  spline S11 degree 5 poles (11.9856, 0.5875) (11.9781, 0.5928) (11.9632, 0.6035) (11.9408, 0.6194) (11.9109, 0.6405) (11.8733, 0.6665) (11.8358, 0.6923) (11.7981, 0.7177) (11.7603, 0.7429) (11.7225, 0.7677) (11.6846, 0.7923) (11.6466, 0.8166) (11.6085, 0.8406) (11.5704, 0.8642) (11.5322, 0.8876) (11.4939, 0.9107) (11.4556, 0.9334) (11.4172, 0.9559) (11.3787, 0.978) (11.3402, 0.9998) (11.3016, 1.0213) (11.2629, 1.0425) (11.2242, 1.0634) (11.1855, 1.084) (11.1466, 1.1042) (11.1078, 1.1241) (11.0688, 1.1437) (11.0298, 1.1629) (10.9908, 1.1818) (10.9517, 1.2004) (10.9126, 1.2187) (10.8734, 1.2366) (10.8342, 1.2541) (10.795, 1.2713) (10.7557, 1.2882) (10.7163, 1.3047) (10.677, 1.3209) (10.6376, 1.3367) (10.5982, 1.3521) (10.5587, 1.3672) (10.5192, 1.3819) (10.4797, 1.3962) (10.4402, 1.4102) (10.4006, 1.4237) (10.3611, 1.4369) (10.3215, 1.4497) (10.2819, 1.4621) (10.2423, 1.4741) (10.2027, 1.4857) (10.163, 1.4969) (10.1234, 1.5076) (10.0838, 1.5179) (10.0441, 1.5278) (10.0045, 1.5372) (9.9649, 1.5461) (9.9253, 1.5546) (9.8857, 1.5626) (9.8461, 1.5702) (9.8065, 1.5774) (9.767, 1.5842) (9.7275, 1.5903) (9.688, 1.5957) (9.6485, 1.6005) (9.6092, 1.6044) (9.5699, 1.6078) (9.5306, 1.6106) (9.4913, 1.6131) (9.4522, 1.6153) (9.4131, 1.6169) (9.374, 1.6176) (9.3352, 1.6169) (9.3043, 1.6147) (9.2813, 1.6119) (9.2659, 1.6095) (9.2583, 1.6082) knots -1 -1 -1 -1 -1 -1 -0.98571429 -0.97142857 -0.95714286 -0.94285714 -0.92857143 -0.91428571 -0.9 -0.88571429 -0.87142857 -0.85714286 -0.84285714 -0.82857143 -0.81428571 -0.8 -0.78571429 -0.77142857 -0.75714286 -0.74285714 -0.72857143 -0.71428571 -0.7 -0.68571429 -0.67142857 -0.65714286 -0.64285714 -0.62857143 -0.61428571 -0.6 -0.58571429 -0.57142857 -0.55714286 -0.54285714 -0.52857143 -0.51428571 -0.5 -0.48571429 -0.47142857 -0.45714286 -0.44285714 -0.42857143 -0.41428571 -0.4 -0.38571429 -0.37142857 -0.35714286 -0.34285714 -0.32857143 -0.31428571 -0.3 -0.28571429 -0.27142857 -0.25714286 -0.24285714 -0.22857143 -0.21428571 -0.2 -0.18571429 -0.17142857 -0.15714286 -0.14285714 -0.12857143 -0.11428571 -0.1 -0.08571429 -0.07142857 -0.05714286 -0.04285714 -0.02857143 -0.01428571 0 0 0 0 0 0
  line L11 (9.2583, 1.6082) -> (8.3641, 1.4537)
  arc A23 (7.2354, 2.1538) -> (8.3641, 1.4537) centre (8.1939, 2.4391) ccw
  arc A24 (7.2354, 2.1538) -> (7.1196, 2.5104) centre (0, 0) ccw
  arc A25 (7.6212, 3.7403) -> (7.1196, 2.5104) centre (8.0626, 2.843) ccw
  line L12 (7.6212, 3.7403) -> (8.4354, 4.1409)
  spline S12 degree 5 poles (8.4354, 4.1409) (8.4423, 4.1443) (8.4561, 4.1514) (8.4764, 4.1627) (8.5027, 4.179) (8.5346, 4.2013) (8.5657, 4.2248) (8.5964, 4.2491) (8.6268, 4.2738) (8.6571, 4.2989) (8.6872, 4.3243) (8.7171, 4.3501) (8.7466, 4.3765) (8.7757, 4.4035) (8.8044, 4.4311) (8.8328, 4.4593) (8.8608, 4.4879) (8.8886, 4.517) (8.9162, 4.5465) (8.9435, 4.5763) (8.9705, 4.6064) (8.9973, 4.6369) (9.0239, 4.6678) (9.0502, 4.699) (9.0762, 4.7307) (9.1019, 4.7627) (9.1274, 4.795) (9.1526, 4.8277) (9.1776, 4.8607) (9.2024, 4.894) (9.2269, 4.9276) (9.2511, 4.9615) (9.2752, 4.9957) (9.299, 5.0303) (9.3225, 5.0651) (9.3458, 5.1002) (9.3688, 5.1356) (9.3917, 5.1712) (9.4142, 5.2072) (9.4366, 5.2434) (9.4587, 5.2799) (9.4806, 5.3166) (9.5022, 5.3536) (9.5236, 5.3908) (9.5448, 5.4283) (9.5657, 5.4661) (9.5864, 5.5041) (9.6069, 5.5424) (9.6271, 5.5808) (9.6471, 5.6196) (9.6668, 5.6585) (9.6864, 5.6977) (9.7056, 5.7371) (9.7247, 5.7768) (9.7435, 5.8166) (9.7621, 5.8567) (9.7804, 5.897) (9.7986, 5.9376) (9.8164, 5.9783) (9.8341, 6.0192) (9.8515, 6.0604) (9.8686, 6.1017) (9.8856, 6.1433) (9.9023, 6.1851) (9.9187, 6.227) (9.935, 6.2692) (9.951, 6.3115) (9.9667, 6.3541) (9.9822, 6.3968) (9.9975, 6.4398) (10.0126, 6.4829) (10.0244, 6.5175) (10.0332, 6.5436) (10.039, 6.561) (10.0419, 6.5697) knots 0 0 0 0 0 0 0.01428571 0.02857143 0.04285714 0.05714286 0.07142857 0.08571429 0.1 0.11428571 0.12857143 0.14285714 0.15714286 0.17142857 0.18571429 0.2 0.21428571 0.22857143 0.24285714 0.25714286 0.27142857 0.28571429 0.3 0.31428571 0.32857143 0.34285714 0.35714286 0.37142857 0.38571429 0.4 0.41428571 0.42857143 0.44285714 0.45714286 0.47142857 0.48571429 0.5 0.51428571 0.52857143 0.54285714 0.55714286 0.57142857 0.58571429 0.6 0.61428571 0.62857143 0.64285714 0.65714286 0.67142857 0.68571429 0.7 0.71428571 0.72857143 0.74285714 0.75714286 0.77142857 0.78571429 0.8 0.81428571 0.82857143 0.84285714 0.85714286 0.87142857 0.88571429 0.9 0.91428571 0.92857143 0.94285714 0.95714286 0.97142857 0.98571429 1 1 1 1 1 1
  arc A26 (10.0419, 6.5697) -> (9.3513, 7.5202) centre (0, 0) ccw
  spline S13 degree 5 poles (9.3513, 7.5202) (9.3421, 7.5202) (9.3237, 7.52) (9.2962, 7.5198) (9.2596, 7.5192) (9.214, 7.5182) (9.1684, 7.5169) (9.123, 7.5154) (9.0777, 7.5136) (9.0324, 7.5114) (8.9873, 7.509) (8.9423, 7.5063) (8.8974, 7.5034) (8.8527, 7.5001) (8.808, 7.4965) (8.7635, 7.4927) (8.7191, 7.4886) (8.6749, 7.4842) (8.6307, 7.4795) (8.5867, 7.4745) (8.5429, 7.4692) (8.4991, 7.4636) (8.4555, 7.4577) (8.4121, 7.4516) (8.3688, 7.4451) (8.3256, 7.4384) (8.2826, 7.4313) (8.2398, 7.424) (8.1971, 7.4164) (8.1545, 7.4084) (8.1122, 7.4002) (8.07, 7.3916) (8.0279, 7.3828) (7.986, 7.3737) (7.9443, 7.3642) (7.9028, 7.3544) (7.8615, 7.3444) (7.8203, 7.334) (7.7793, 7.3233) (7.7386, 7.3123) (7.698, 7.301) (7.6576, 7.2894) (7.6174, 7.2774) (7.5775, 7.2652) (7.5377, 7.2526) (7.4982, 7.2396) (7.4588, 7.2264) (7.4197, 7.2128) (7.3809, 7.1989) (7.3422, 7.1847) (7.3038, 7.1701) (7.2657, 7.1551) (7.2279, 7.1398) (7.1903, 7.1241) (7.153, 7.108) (7.116, 7.0916) (7.0792, 7.0748) (7.0427, 7.0577) (7.0064, 7.0403) (6.9705, 7.0225) (6.9349, 7.0042) (6.8998, 6.9854) (6.8651, 6.9661) (6.8309, 6.9462) (6.7971, 6.9257) (6.7637, 6.905) (6.7305, 6.8839) (6.6975, 6.8626) (6.6649, 6.8409) (6.633, 6.8186) (6.602, 6.7952) (6.5783, 6.7752) (6.5613, 6.7594) (6.5503, 6.7485) (6.5449, 6.7429) knots -1 -1 -1 -1 -1 -1 -0.98571429 -0.97142857 -0.95714286 -0.94285714 -0.92857143 -0.91428571 -0.9 -0.88571429 -0.87142857 -0.85714286 -0.84285714 -0.82857143 -0.81428571 -0.8 -0.78571429 -0.77142857 -0.75714286 -0.74285714 -0.72857143 -0.71428571 -0.7 -0.68571429 -0.67142857 -0.65714286 -0.64285714 -0.62857143 -0.61428571 -0.6 -0.58571429 -0.57142857 -0.55714286 -0.54285714 -0.52857143 -0.51428571 -0.5 -0.48571429 -0.47142857 -0.45714286 -0.44285714 -0.42857143 -0.41428571 -0.4 -0.38571429 -0.37142857 -0.35714286 -0.34285714 -0.32857143 -0.31428571 -0.3 -0.28571429 -0.27142857 -0.25714286 -0.24285714 -0.22857143 -0.21428571 -0.2 -0.18571429 -0.17142857 -0.15714286 -0.14285714 -0.12857143 -0.11428571 -0.1 -0.08571429 -0.07142857 -0.05714286 -0.04285714 -0.02857143 -0.01428571 0 0 0 0 0 0
  line L13 (6.5449, 6.7429) -> (5.9123, 6.0924)
  arc A27 (4.5876, 5.9953) -> (5.9123, 6.0924) centre (5.1953, 6.7895) ccw
  arc A28 (4.5876, 5.9953) -> (4.2842, 6.2158) centre (0, 0) ccw
  arc A29 (3.9672, 7.5055) -> (4.2842, 6.2158) centre (4.8518, 7.0391) ccw
  line L14 (3.9672, 7.5055) -> (4.3904, 8.3082)
  spline S14 degree 5 poles (4.3904, 8.3082) (4.394, 8.3151) (4.401, 8.3289) (4.4108, 8.35) (4.4225, 8.3787) (4.4352, 8.4154) (4.4465, 8.4527) (4.4571, 8.4904) (4.4672, 8.5283) (4.4769, 8.5664) (4.4863, 8.6046) (4.4953, 8.6431) (4.5037, 8.6817) (4.5114, 8.7207) (4.5184, 8.7599) (4.5248, 8.7994) (4.5306, 8.8391) (4.536, 8.879) (4.541, 8.919) (4.5455, 8.9591) (4.5497, 8.9994) (4.5535, 9.0398) (4.5568, 9.0804) (4.5597, 9.1212) (4.5621, 9.162) (4.5641, 9.2031) (4.5657, 9.2442) (4.567, 9.2855) (4.5678, 9.3269) (4.5682, 9.3683) (4.5683, 9.4099) (4.568, 9.4516) (4.5673, 9.4934) (4.5663, 9.5353) (4.5649, 9.5773) (4.5631, 9.6194) (4.5609, 9.6616) (4.5584, 9.7039) (4.5556, 9.7462) (4.5524, 9.7887) (4.5488, 9.8312) (4.5449, 9.8738) (4.5407, 9.9164) (4.5361, 9.9591) (4.5312, 10.0019) (4.5259, 10.0448) (4.5203, 10.0877) (4.5144, 10.1306) (4.5081, 10.1737) (4.5016, 10.2167) (4.4946, 10.2599) (4.4874, 10.303) (4.4798, 10.3463) (4.4719, 10.3895) (4.4637, 10.4329) (4.4552, 10.4762) (4.4464, 10.5196) (4.4372, 10.563) (4.4277, 10.6065) (4.4179, 10.65) (4.4078, 10.6935) (4.3974, 10.7371) (4.3867, 10.7806) (4.3756, 10.8242) (4.3643, 10.8679) (4.3526, 10.9115) (4.3407, 10.9552) (4.3284, 10.9989) (4.3158, 11.0426) (4.303, 11.0863) (4.2898, 11.13) (4.279, 11.165) (4.2708, 11.1912) (4.2653, 11.2087) (4.2625, 11.2175) knots 0 0 0 0 0 0 0.01428571 0.02857143 0.04285714 0.05714286 0.07142857 0.08571429 0.1 0.11428571 0.12857143 0.14285714 0.15714286 0.17142857 0.18571429 0.2 0.21428571 0.22857143 0.24285714 0.25714286 0.27142857 0.28571429 0.3 0.31428571 0.32857143 0.34285714 0.35714286 0.37142857 0.38571429 0.4 0.41428571 0.42857143 0.44285714 0.45714286 0.47142857 0.48571429 0.5 0.51428571 0.52857143 0.54285714 0.55714286 0.57142857 0.58571429 0.6 0.61428571 0.62857143 0.64285714 0.65714286 0.67142857 0.68571429 0.7 0.71428571 0.72857143 0.74285714 0.75714286 0.77142857 0.78571429 0.8 0.81428571 0.82857143 0.84285714 0.85714286 0.87142857 0.88571429 0.9 0.91428571 0.92857143 0.94285714 0.95714286 0.97142857 0.98571429 1 1 1 1 1 1
  arc A30 (4.2625, 11.2175) -> (3.145, 11.5805) centre (0, 0) ccw
  spline S15 degree 5 poles (3.145, 11.5805) (3.1376, 11.5751) (3.1229, 11.5642) (3.1008, 11.5478) (3.0715, 11.5258) (3.0352, 11.4982) (2.9991, 11.4704) (2.9632, 11.4424) (2.9276, 11.4143) (2.8923, 11.386) (2.8572, 11.3575) (2.8224, 11.3289) (2.7878, 11.3001) (2.7535, 11.2712) (2.7195, 11.2421) (2.6857, 11.2128) (2.6522, 11.1834) (2.619, 11.1538) (2.5861, 11.124) (2.5534, 11.0941) (2.521, 11.0641) (2.4889, 11.0339) (2.4571, 11.0035) (2.4256, 10.973) (2.3944, 10.9423) (2.3634, 10.9115) (2.3328, 10.8805) (2.3024, 10.8494) (2.2724, 10.8181) (2.2426, 10.7867) (2.2132, 10.7551) (2.184, 10.7234) (2.1552, 10.6915) (2.1267, 10.6595) (2.0985, 10.6273) (2.0707, 10.595) (2.0431, 10.5626) (2.0159, 10.53) (1.9891, 10.4973) (1.9625, 10.4644) (1.9364, 10.4314) (1.9105, 10.3983) (1.885, 10.365) (1.8599, 10.3316) (1.8352, 10.298) (1.8108, 10.2643) (1.7868, 10.2305) (1.7631, 10.1965) (1.7398, 10.1624) (1.7169, 10.1282) (1.6945, 10.0938) (1.6724, 10.0593) (1.6508, 10.0246) (1.6296, 9.9899) (1.6089, 9.9549) (1.5886, 9.9199) (1.5687, 9.8847) (1.5492, 9.8494) (1.5301, 9.814) (1.5115, 9.7785) (1.4935, 9.7428) (1.4761, 9.7069) (1.4594, 9.6709) (1.4435, 9.6347) (1.4282, 9.5983) (1.4133, 9.5618) (1.3988, 9.5253) (1.3847, 9.4887) (1.371, 9.452) (1.3583, 9.4151) (1.347, 9.378) (1.3396, 9.3479) (1.3351, 9.3251) (1.3326, 9.3098) (1.3315, 9.3021) knots -1 -1 -1 -1 -1 -1 -0.98571429 -0.97142857 -0.95714286 -0.94285714 -0.92857143 -0.91428571 -0.9 -0.88571429 -0.87142857 -0.85714286 -0.84285714 -0.82857143 -0.81428571 -0.8 -0.78571429 -0.77142857 -0.75714286 -0.74285714 -0.72857143 -0.71428571 -0.7 -0.68571429 -0.67142857 -0.65714286 -0.64285714 -0.62857143 -0.61428571 -0.6 -0.58571429 -0.57142857 -0.55714286 -0.54285714 -0.52857143 -0.51428571 -0.5 -0.48571429 -0.47142857 -0.45714286 -0.44285714 -0.42857143 -0.41428571 -0.4 -0.38571429 -0.37142857 -0.35714286 -0.34285714 -0.32857143 -0.31428571 -0.3 -0.28571429 -0.27142857 -0.25714286 -0.24285714 -0.22857143 -0.21428571 -0.2 -0.18571429 -0.17142857 -0.15714286 -0.14285714 -0.12857143 -0.11428571 -0.1 -0.08571429 -0.07142857 -0.05714286 -0.04285714 -0.02857143 -0.01428571 0 0 0 0 0 0
  line L15 (1.3315, 9.3021) -> (1.2021, 8.404)
  arc A31 (0.1875, 7.5469) -> (1.2021, 8.404) centre (0.2123, 8.5466) ccw
  arc A32 (0.1875, 7.5469) -> (-0.1875, 7.5469) centre (0, 0) ccw
  arc A33 (-1.2021, 8.404) -> (-0.1875, 7.5469) centre (-0.2123, 8.5466) ccw
  line L16 (-1.2021, 8.404) -> (-1.3315, 9.3021)
  spline S16 degree 5 poles (-1.3315, 9.3021) (-1.3326, 9.3098) (-1.3351, 9.3251) (-1.3396, 9.3479) (-1.347, 9.378) (-1.3583, 9.4151) (-1.371, 9.452) (-1.3847, 9.4887) (-1.3988, 9.5253) (-1.4133, 9.5618) (-1.4282, 9.5983) (-1.4435, 9.6347) (-1.4594, 9.6709) (-1.4761, 9.7069) (-1.4935, 9.7428) (-1.5115, 9.7785) (-1.5301, 9.814) (-1.5492, 9.8494) (-1.5687, 9.8847) (-1.5886, 9.9199) (-1.6089, 9.9549) (-1.6296, 9.9899) (-1.6508, 10.0246) (-1.6724, 10.0593) (-1.6945, 10.0938) (-1.7169, 10.1282) (-1.7398, 10.1624) (-1.7631, 10.1965) (-1.7868, 10.2305) (-1.8108, 10.2643) (-1.8352, 10.298) (-1.8599, 10.3316) (-1.885, 10.365) (-1.9105, 10.3983) (-1.9364, 10.4314) (-1.9625, 10.4644) (-1.9891, 10.4973) (-2.0159, 10.53) (-2.0431, 10.5626) (-2.0707, 10.595) (-2.0985, 10.6273) (-2.1267, 10.6595) (-2.1552, 10.6915) (-2.184, 10.7234) (-2.2132, 10.7551) (-2.2426, 10.7867) (-2.2724, 10.8181) (-2.3024, 10.8494) (-2.3328, 10.8805) (-2.3634, 10.9115) (-2.3944, 10.9423) (-2.4256, 10.973) (-2.4571, 11.0035) (-2.4889, 11.0339) (-2.521, 11.0641) (-2.5534, 11.0941) (-2.5861, 11.124) (-2.619, 11.1538) (-2.6522, 11.1834) (-2.6857, 11.2128) (-2.7195, 11.2421) (-2.7535, 11.2712) (-2.7878, 11.3001) (-2.8224, 11.3289) (-2.8572, 11.3575) (-2.8923, 11.386) (-2.9276, 11.4143) (-2.9632, 11.4424) (-2.9991, 11.4704) (-3.0352, 11.4982) (-3.0715, 11.5258) (-3.1008, 11.5478) (-3.1229, 11.5642) (-3.1376, 11.5751) (-3.145, 11.5805) knots 0 0 0 0 0 0 0.01428571 0.02857143 0.04285714 0.05714286 0.07142857 0.08571429 0.1 0.11428571 0.12857143 0.14285714 0.15714286 0.17142857 0.18571429 0.2 0.21428571 0.22857143 0.24285714 0.25714286 0.27142857 0.28571429 0.3 0.31428571 0.32857143 0.34285714 0.35714286 0.37142857 0.38571429 0.4 0.41428571 0.42857143 0.44285714 0.45714286 0.47142857 0.48571429 0.5 0.51428571 0.52857143 0.54285714 0.55714286 0.57142857 0.58571429 0.6 0.61428571 0.62857143 0.64285714 0.65714286 0.67142857 0.68571429 0.7 0.71428571 0.72857143 0.74285714 0.75714286 0.77142857 0.78571429 0.8 0.81428571 0.82857143 0.84285714 0.85714286 0.87142857 0.88571429 0.9 0.91428571 0.92857143 0.94285714 0.95714286 0.97142857 0.98571429 1 1 1 1 1 1
  arc A34 (-3.145, 11.5805) -> (-4.2625, 11.2175) centre (0, 0) ccw
  spline S17 degree 5 poles (-4.2625, 11.2175) (-4.2653, 11.2087) (-4.2708, 11.1912) (-4.279, 11.165) (-4.2898, 11.13) (-4.303, 11.0863) (-4.3158, 11.0426) (-4.3284, 10.9989) (-4.3407, 10.9552) (-4.3526, 10.9115) (-4.3643, 10.8679) (-4.3756, 10.8242) (-4.3867, 10.7806) (-4.3974, 10.7371) (-4.4078, 10.6935) (-4.4179, 10.65) (-4.4277, 10.6065) (-4.4372, 10.563) (-4.4464, 10.5196) (-4.4552, 10.4762) (-4.4637, 10.4329) (-4.4719, 10.3895) (-4.4798, 10.3463) (-4.4874, 10.303) (-4.4946, 10.2599) (-4.5016, 10.2167) (-4.5081, 10.1737) (-4.5144, 10.1306) (-4.5203, 10.0877) (-4.5259, 10.0448) (-4.5312, 10.0019) (-4.5361, 9.9591) (-4.5407, 9.9164) (-4.5449, 9.8738) (-4.5488, 9.8312) (-4.5524, 9.7887) (-4.5556, 9.7462) (-4.5584, 9.7039) (-4.5609, 9.6616) (-4.5631, 9.6194) (-4.5649, 9.5773) (-4.5663, 9.5353) (-4.5673, 9.4934) (-4.568, 9.4516) (-4.5683, 9.4099) (-4.5682, 9.3683) (-4.5678, 9.3269) (-4.567, 9.2855) (-4.5657, 9.2442) (-4.5641, 9.2031) (-4.5621, 9.162) (-4.5597, 9.1212) (-4.5568, 9.0804) (-4.5535, 9.0398) (-4.5497, 8.9994) (-4.5455, 8.9591) (-4.541, 8.919) (-4.536, 8.879) (-4.5306, 8.8391) (-4.5248, 8.7994) (-4.5184, 8.7599) (-4.5114, 8.7207) (-4.5037, 8.6817) (-4.4953, 8.6431) (-4.4863, 8.6046) (-4.4769, 8.5664) (-4.4672, 8.5283) (-4.4571, 8.4904) (-4.4465, 8.4527) (-4.4352, 8.4154) (-4.4225, 8.3787) (-4.4108, 8.35) (-4.401, 8.3289) (-4.394, 8.3151) (-4.3904, 8.3082) knots -1 -1 -1 -1 -1 -1 -0.98571429 -0.97142857 -0.95714286 -0.94285714 -0.92857143 -0.91428571 -0.9 -0.88571429 -0.87142857 -0.85714286 -0.84285714 -0.82857143 -0.81428571 -0.8 -0.78571429 -0.77142857 -0.75714286 -0.74285714 -0.72857143 -0.71428571 -0.7 -0.68571429 -0.67142857 -0.65714286 -0.64285714 -0.62857143 -0.61428571 -0.6 -0.58571429 -0.57142857 -0.55714286 -0.54285714 -0.52857143 -0.51428571 -0.5 -0.48571429 -0.47142857 -0.45714286 -0.44285714 -0.42857143 -0.41428571 -0.4 -0.38571429 -0.37142857 -0.35714286 -0.34285714 -0.32857143 -0.31428571 -0.3 -0.28571429 -0.27142857 -0.25714286 -0.24285714 -0.22857143 -0.21428571 -0.2 -0.18571429 -0.17142857 -0.15714286 -0.14285714 -0.12857143 -0.11428571 -0.1 -0.08571429 -0.07142857 -0.05714286 -0.04285714 -0.02857143 -0.01428571 0 0 0 0 0 0
  line L17 (-4.3904, 8.3082) -> (-3.9672, 7.5055)
  arc A35 (-4.2842, 6.2158) -> (-3.9672, 7.5055) centre (-4.8518, 7.0391) ccw
  arc A36 (-4.2842, 6.2158) -> (-4.5876, 5.9953) centre (0, 0) ccw
  arc A37 (-5.9123, 6.0924) -> (-4.5876, 5.9953) centre (-5.1953, 6.7895) ccw
  line L18 (-5.9123, 6.0924) -> (-6.5449, 6.7429)